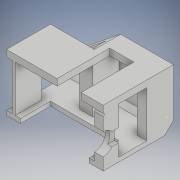
# Autodesk Inventor part: Basev3.3
Saved by Autodesk Inventor 2018 (Build 220112000, 112)
## iProperties
Created: 2017-07-13
Part Number: Basev3.3
Material: Generic
Document SubType Name: Modeling
Designer: JAck
Density: 1 g/cm^3
Appearance: Default
Author: JAck
Autodesk Inventor part; units mm, degrees
ref_plane "YZ Plane" through (0, 0, 0) normal (1, 0, 0) x (0, 1, 0)
ref_plane "XZ Plane" through (0, 0, 0) normal (0, 1, 0) x (-1, 0, 0)
ref_plane "XY Plane" through (0, 0, 0) normal (0, 0, 1) x (1, 0, 0)
sketch "Sketch1" plane through (0, 0, 0) normal (0, 1, 0) x (-1, 0, 0)
  line L0 (48.2977, 71.5211) -> (-16.7023, 71.5211)
  line L1 (-16.7023, 71.5211) -> (-16.7023, -8.4789)
  line L2 (-16.7023, -8.4789) -> (48.2977, -8.4789)
  line L3 (48.2977, -8.4789) -> (48.2977, 71.5211)
  arc A0 (22.2975, -8.4789) -> (-2.7023, -8.4789) centre (9.7976, -8.4281) ccw
  line L4 (-16.7023, -8.4789) -> (-11.7023, -8.4789)
  line L5 (-11.7023, -8.4789) -> (-11.7023, 71.5211)
  line L6 (-11.7023, 71.5211) -> (-16.7023, 71.5211)
  line L7 (-16.7023, 71.5211) -> (-16.7023, -8.4789)
  line L8 (48.2977, -8.4789) -> (40.7977, -8.4789)
  line L9 (40.7977, -8.4789) -> (40.7977, 71.5211)
  line L10 (40.7977, 71.5211) -> (48.2977, 71.5211)
  line L11 (48.2977, 71.5211) -> (48.2977, -8.4789)
  line L12 (-11.7023, -8.4789) -> (40.7977, -8.4789)
  line L13 (40.7977, -8.4789) -> (40.7977, 9.0211)
  line L14 (40.7977, 9.0211) -> (-11.7023, 9.0211)
  line L15 (-11.7023, 9.0211) -> (-11.7023, -8.4789)
  line L16 (-11.7023, 71.5211) -> (40.7977, 71.5211)
  line L17 (40.7977, 71.5211) -> (40.7977, 64.0211)
  line L18 (40.7977, 64.0211) -> (-11.7023, 64.0211)
  line L19 (-11.7023, 64.0211) -> (-11.7023, 71.5211)
  line L20 (-16.7023, 61.5211) -> (-6.7023, 71.5211)
  line L21 (-16.7023, 61.5211) -> (-16.7023, 71.5211)
  line L22 (-6.7023, 71.5211) -> (-11.7023, 66.5211)
  line L23 (-11.7023, 64.0211) -> (-11.7023, 66.5211)
  line L24 (-6.7023, 71.5211) -> (40.7977, 71.5211)
  line L25 (40.7977, 64.0211) -> (-11.7023, 64.0211)
  line L26 (-11.7023, 66.5211) -> (-11.7023, 64.0211)
  line L27 (-11.7023, 66.5211) -> (-6.7023, 71.5211)
  line L28 (-11.7023, 54.0211) -> (-1.7023, 64.0211)
  point P0 (0, 0)
  dimension "d0" = 80
  dimension "d1" = 65
  dimension "d3" = 14
  dimension "d4" = 12.5
  dimension "d5" = 7.5
  dimension "d6" = 5
  dimension "d7" = 17.5
  dimension "d8" = 7.5
  dimension "d9" = 10
  dimension "d10" = 10
  dimension "d48" = 10
  dimension "d49" = 10
  constraints: 58 end point, 11 parallel, 11 point on line, 6 perpendicular, 5 horizontal, 4 collinear, 2 point on circle, 1 centre point, 1 midpoint
  measures "d0" distance of L2.end L0.start
  measures "d1" distance of L1.end L2.end
  measures "d3" distance from line of L1 A0.end
  measures "d4" radius of A0
  measures "d5" distance between parallel lines of L3 L9
  measures "d6" distance between parallel lines of L5 L1
  measures "d7" distance between parallel lines of L2 L14
  measures "d8" distance between parallel lines of L18 L0
  measures "d9" distance from line of L0 L20.start
  measures "d10" distance from line of L1 L20.end
  measures "d48" distance of L18.end L28.start
  measures "d49" distance of L18.end L28.end
extrude "Extrusion1" add sketch "Sketch1" along normal blind 110 contours L3 L2 L9 L0 | L9 L18 L5 L20 L0 | L2 A0 L5 L14 L9 | L5 L2 L1 L20
sketch "Sketch2" plane through (-22.2975, 0, -8.4789) normal (0, 0, -1) x (-1, 0, 0)
  line L0 (18.5002, 0) -> (18.5002, 110) projected
  line L1 (18.5002, 110) -> (-33.9998, 110)
  line L2 (-33.9998, 110) -> (-33.9998, 10)
  line L3 (-33.9998, 10) -> (18.5002, 10)
  line L4 (18.5002, 10) -> (18.5002, 110)
  point P0 (-22.2975, 0)
  dimension "d13" = 100
  dimension "d14" = 52.5
  constraints: 8 end point, 2 parallel, 1 horizontal, 1 perpendicular
  measures "d13" distance between parallel lines of L3 L1
  measures "d14" distance between parallel lines of L0 L2
extrude "Extrusion2" cut sketch "Sketch2" against normal blind 30
sketch "Sketch3" plane through (-40.7977, 0, 9.0211) normal (0, 0, 1) x (1, 0, 0)
  line L0 (52.5, 10) -> (0, 10) projected
  line L1 (26.0002, 10) -> (36, 10)
  line L2 (18.5002, 10) -> (18.5002, 0) projected
  line L3 (43.5, 0) -> (43.5, 10) projected
  line L4 (0, 0) -> (52.5, 0) projected
  line L5 (38.5, 0) -> (23.5002, 0)
  line L6 (23.5002, 0) -> (23.5002, 5)
  line L7 (23.5002, 5) -> (38.5, 5)
  line L8 (38.5, 5) -> (38.5, 0)
  point P0 (40.7977, 0)
  dimension "d43" = 5
  dimension "d44" = 5
  dimension "d45" = 5
  constraints: 10 end point, 2 horizontal, 2 parallel, 2 point on line, 1 perpendicular
  measures "d43" distance between parallel lines of L3 L8
  measures "d44" distance between parallel lines of L2 L6
  measures "d45" distance between parallel lines of L4 L7
sketch "Sketch4" plane through (16.7023, 0, 61.5211) normal (1, 0, 0) x (0, 0, -1)
  line L0 (70, 110) -> (70, 10) projected
  line L1 (70, 94) -> (36, 94)
  line L2 (36, 94) -> (36, 16)
  line L3 (36, 16) -> (70, 16)
  line L4 (70, 16) -> (70, 94)
  line L5 (0, 0) -> (70, 0) projected
  line L6 (0, 110) -> (70, 110) projected
  point P0 (61.5211, 0)
  dimension "d22" = 34
  dimension "d23" = 16
  dimension "d24" = 16
  dimension "d25" = 78
  constraints: 8 end point, 2 parallel, 1 horizontal, 1 perpendicular, 1 point on line
  measures "d22" distance between parallel lines of L0 L2
  measures "d23" distance between parallel lines of L5 L3
  measures "d24" distance between parallel lines of L6 L1
  measures "d25" distance between parallel lines of L3 L1
extrude "Extrusion4" cut sketch "Sketch4" against normal blind 30
sketch "Sketch5" plane through (0, 0, 0) normal (0, -1, 0) x (1, 0, 0)
  line L0 (-40.7977, -8.4789) -> (-22.2975, -8.4789) projected
  arc A0 (-40.2975, -8.4789) -> (-37.2975, -8.4789) centre (-38.7975, -8.4789) ccw
  arc A1 (-37.2975, -8.4789) -> (-40.2975, -8.4789) centre (-38.7975, -8.4789) ccw
  point P0 (0, 0)
  dimension "d28" = 18
  dimension "d29" = 1.5
  dimension "d30" = 0
  dimension "d31" = 1.5
  constraints: 4 point on circle, 2 centre point, 2 point on line
  measures "d28" distance of L0.end A0.start
  measures "d29" radius of A0
  measures "d30" distance from line of L0 A0.centre
  measures "d31" radius of A1
extrude "Extrusion5" cut sketch "Sketch5" against normal blind 30 contours A1 L0
sketch "Sketch7" plane through (-48.2977, 0, 71.5211) normal (0, 0, 1) x (1, 0, 0)
  line L0 (0, 110) -> (55, 110) projected
  line L1 (0, 110) -> (40, 110)
  line L2 (40, 110) -> (0, 60)
  line L3 (0, 60) -> (0, 110)
  line L4 (65, 110) -> (65, 0) projected
  point P0 (48.2977, 0)
  dimension "d39" = 40
  dimension "d40" = 25
  dimension "d41" = 50
  constraints: 6 end point, 2 point on line, 1 perpendicular
  measures "d39" distance of L1.end L1.start
  measures "d40" distance from line of L4 L1.end
  measures "d41" distance of L2.end L1.start
extrude "Extrusion6" cut sketch "Sketch3" against normal blind 30 contours L4 L6 L7 L8
sketch "Sketch8" plane through (0, 110, 0) normal (0, 1, 0) x (1, 0, 0)
  line L0 (11.7023, 8.4789) -> (11.7023, -64.0211) projected
  line L1 (11.7023, -59.0211) -> (6.7023, -64.0211)
  line L2 (6.7023, -64.0211) -> (11.7023, -64.0211)
  line L3 (11.7023, -64.0211) -> (11.7023, -59.0211)
  point P0 (0, 0)
  dimension "d50" = 5
  dimension "d51" = 5
  constraints: 6 end point, 1 collinear, 1 perpendicular, 1 point on line
  measures "d50" distance of L1.start L0.end
  measures "d51" distance of L0.end L1.end
extrude "Extrusion7" add sketch "Sketch8" against normal up to surface (110 mm away)
extrude "Extrusion8" cut sketch "Sketch7" against normal blind 30
sketch "Sketch9" plane through (11.7023, 0, 9.0211) normal (-1, 0, 0) x (0, 0, 1)
  line L0 (32.5, 69.375) -> (55, 69.375) projected
  line L1 (50, 0) -> (50, 110) projected
  line L2 (50, 69.375) -> (25, 69.375)
  line L3 (25, 69.375) -> (25, 54.375)
  line L4 (25, 54.375) -> (50, 54.375)
  line L5 (50, 54.375) -> (50, 69.375)
  point P0 (-9.0211, 0)
  dimension "d56" = 15
  dimension "d57" = 25
  constraints: 8 end point, 2 parallel, 2 point on line, 1 horizontal, 1 perpendicular
  measures "d56" distance between parallel lines of L4 L0
  measures "d57" distance of L2.start L2.end
sketch "Sketch11" plane through (11.7023, 0, 9.0211) normal (-1, 0, 0) x (0, 0, 1)
  line L0 (-17.5, 94) -> (-17.5, 110) projected
  line L1 (-17.5, 100) -> (12.5, 100)
  line L2 (12.5, 100) -> (12.5, 103.5)
  line L3 (12.5, 103.5) -> (-17.5, 103.5)
  line L4 (-17.5, 103.5) -> (-17.5, 100)
  line L5 (-17.5, 110) -> (50, 110) projected
  point P0 (-9.0211, 0)
  dimension "d62" = 3.5
  dimension "d63" = 30
  dimension "d64" = 10
  constraints: 8 end point, 2 parallel, 1 horizontal, 1 perpendicular, 1 point on line
  measures "d62" distance between parallel lines of L1 L3
  measures "d63" distance between parallel lines of L4 L2
  measures "d64" distance between parallel lines of L5 L1
extrude "Extrusion11" add sketch "Sketch11" along normal up to next
sketch "Sketch12" plane through (-48.2977, 0, -8.4789) normal (-1, 0, 0) x (0, 0, 1)
  line L0 (0, 100) -> (0, 10) projected
  line L1 (0, 52.5) -> (60, 52.5)
  line L2 (60, 52.5) -> (60, 25)
  line L3 (60, 25) -> (0, 25)
  line L4 (0, 25) -> (0, 52.5)
  line L5 (80, 0) -> (80, 60) projected
  line L6 (80, 60) -> (50, 60) projected
  point P0 (8.4789, 0)
  dimension "d67" = 27.5
  dimension "d68" = 60
  dimension "d69" = 20
  dimension "d70" = 7.5
  constraints: 8 end point, 2 parallel, 1 horizontal, 1 perpendicular, 1 point on line
  measures "d67" distance between parallel lines of L1 L3
  measures "d68" distance of L2.end L3.end
  measures "d69" distance between parallel lines of L5 L2
  measures "d70" distance between parallel lines of L1 L6
extrude "Extrusion12" cut sketch "Sketch12" against normal up to surface (60 mm away)
sketch "Sketch13" plane through (11.7023, 0, 9.0211) normal (-1, 0, 0) x (0, 0, 1)
  line L0 (0, 0) -> (50, 0) projected
  line L1 (50, 0) -> (32.154, 0)
  line L2 (32.154, 0) -> (32.154, 10.7503)
  line L3 (32.154, 10.7503) -> (50, 10.7503)
  line L4 (50, 10.7503) -> (50, 0)
  point P0 (-9.0211, 0)
  constraints: 8 end point, 2 parallel, 1 horizontal, 1 perpendicular
sketch "Sketch14" plane through (6.7023, 0, 64.0211) normal (0, 0, -1) x (-1, 0, 0)
  point P0 (6.7023, 0)
extrude "Extrusion13" add sketch "Sketch9" along normal up to next
extrude "Extrusion14" add sketch "Sketch13" along normal up to next
sketch "Sketch15" plane through (-40.7977, 0, 59.0211) normal (0, 0, 1) x (1, 0, 0)
  line L0 (0, 0) -> (0, 10.7503) projected
  line L1 (52.5, 0) -> (0, 0) projected
  line L2 (52.5, 0) -> (52.5, 10.7503) projected
  line L3 (52.5, 10.7503) -> (0, 10.7503) projected
  line L4 (52.5, 0) -> (52.5, 10.7503) projected
  line L5 (52.5, 0) -> (0, 0) projected
  line L6 (0, 54.375) -> (0, 69.375) projected
  line L7 (52.5, 54.375) -> (0, 54.375) projected
  line L8 (52.5, 54.375) -> (52.5, 69.375) projected
  line L9 (52.5, 69.375) -> (0, 69.375) projected
  point P0 (40.7977, 0)
extrude "Extrusion15" add sketch "Sketch15" along normal blind 5.5
equation "\"d8\" = d5"
equation "\"d49\" = d48"
equation "\"d44\" = d43"
equation "\"d24\" = d23"
equation "\"d31\" = d29"
equation "\"d50\" = d51"
body "Solid1"
